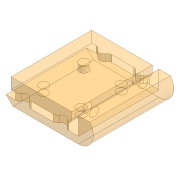
# Autodesk Inventor part: flange7-tip
Saved by Autodesk Inventor 2021 (Build 250183000, 183)
## iProperties
Created: 2022-10-18
Part Number: flange7-tip
Material: Rubber, Silicone
Document SubType Name: Modeling
Designer: alyn649
Density: 1.25 g/cm^3
Appearance: Clear - Yellow(1)
Author: alyn649
Autodesk Inventor part; units mm, degrees
ref_plane "YZ Plane" through (0, 0, 0) normal (1, 0, 0) x (0, 1, 0)
ref_plane "XZ Plane" through (0, 0, 0) normal (0, 1, 0) x (-1, 0, 0)
ref_plane "XY Plane" through (0, 0, 0) normal (0, 0, 1) x (1, 0, 0)
sketch "Sketch2" plane through (0, 0, 0) normal (0, 0, 1) x (1, 0, 0)
  line L0 (-8.072, 0) -> (8.072, 0)
  line L1 (8.072, -1.5) -> (-6.5187, -1.5)
  line L2 (-6.5187, -1.5) -> (-8.072, 0)
  line L3 (-8.8153, 7.7377) -> (-16.0231, 7.7377) construction
  line L4 (8.072, 0) -> (19.7494, 0) construction
  line L5 (8.072, 4) -> (8.072, 0)
  line L6 (8.072, 4) -> (12.608, 4) construction
  arc A0 (8.072, -1.5) -> (10.608, 4) centre (8.072, 1.8347) ccw
  line L7 (10.608, 4) -> (8.072, 4)
  point P0 (0, 0)
  point P1 (0, 0)
  dimension "d0" = 16.144
  dimension "d1" = 136
  dimension "d3" = 1.5
  dimension "d24" = 4
  dimension "d25" = 4.536
  dimension "d26" = 2
  constraints: 16 end point, 4 horizontal, 3 point on circle, 1 centre point, 1 coincident, 1 collinear, 1 midpoint, 1 parallel, 1 point on line, 1 tangent, 1 vertical, 1 vertical alignment
  measures "d0" distance of L0.start L0.end
  measures "d1" angle of L2 L3
  measures "d3" distance between parallel lines of L0 L1
  measures "d24" distance of L5.start L0.end
  measures "d25" distance of L5.start L6.end
  measures "d26" distance of L6.end A0.end
extrude "Extrusion1" add sketch "Sketch2" along normal mid plane 18
sketch "Sketch3" plane through (-8.072, 0, 9) normal (0, 1, 0) x (1, 0, 0)
  circle A0 centre (3.866, 13.5) radius 1
  line L0 (0, 18) -> (16.144, 18) construction
  circle A1 centre (3.866, 18) radius 1 construction
  arc A2 (3, 17.5) -> (2.1339, 18) centre (2.1339, 17) ccw
  arc A3 (3, 17.5) -> (4.732, 17.5) centre (3.866, 18) ccw
  arc A4 (5.5981, 18) -> (4.732, 17.5) centre (5.5981, 17) ccw
  line L1 (2.1339, 18) -> (8.6251, 18) construction
  line L2 (0, 18) -> (0, 0) projected
  line L3 (5.5981, 18) -> (2.1339, 18)
  circle A5 centre (12.279, 13.5) radius 1
  arc A6 (11.413, 17.5) -> (10.5469, 18) centre (10.5469, 17) ccw
  arc A7 (11.413, 17.5) -> (13.145, 17.5) centre (12.279, 18) ccw
  arc A8 (14.0111, 18) -> (13.145, 17.5) centre (14.0111, 17) ccw
  line L4 (14.0111, 18) -> (10.5469, 18)
  line L5 (10.5469, 18) -> (17.0381, 18) construction
  point P0 (8.072, 9)
  point P1 (5.5981, 18)
  point P2 (12.279, 18)
  dimension "d7" = 4.5
  dimension "d8" = 2
  dimension "d9" = 2
  dimension "d10" = 1
  dimension "d11" = 1
  dimension "d23" = 3.866
  dimension "d29" = 8.413
  constraints: 14 point on circle, 9 centre point, 8 end point, 8 tangent, 4 point on line, 1 collinear, 1 horizontal, 1 vertical alignment, 16 other
  measures "d7" vertical distance of A0.centre point (8.072, 9)
  measures "d8" diameter of A1
  measures "d9" diameter of A0
  measures "d10" radius of A2
  measures "d11" radius of A4
  measures "d23" distance from line of L2 A0.centre
  measures "d29" distance of A0.centre A5.centre
extrude "Extrusion2" add sketch "Sketch3" along normal blind 1.5
sketch "Sketch6" plane through (8.072, 4, -9) normal (-1, 0, 0) x (0, 0, 1)
  circle A0 centre (3.5, -1) radius 1
  line L0 (0, 0) -> (18, 0) projected
  line L1 (5.5, -2.5) -> (3.5, -2.5) projected
  point P0 (9, -4)
  point P1 (4.5, -2.5)
  dimension "d35" = 2
  dimension "d36" = 1
  constraints: 1 centre point, 1 midpoint, 1 tangent
  measures "d35" diameter of A0
  measures "d36" horizontal distance of point (4.5, -2.5) A0.centre
extrude "Extrusion5" add sketch "Sketch6" along normal blind 1.5
sketch "Sketch7" plane through (0, 0, -9) normal (0, 0, -1) x (-1, 0, 0)
  line L0 (-8.072, 4) -> (-10.608, 4) construction
  arc A0 (-10.608, 4) -> (-8.072, -1.5) centre (-8.072, 1.8347) ccw construction
  line L1 (-8.072, -1.5) -> (6.5187, -1.5) construction
  line L2 (6.5187, -1.5) -> (8.072, 0) construction
  line L3 (8.072, 0) -> (5.9381, 0) construction
  line L4 (5.9381, 0) -> (5.9381, 1.5) construction
  line L5 (2.4739, 1.5) -> (5.9381, 1.5) construction
  line L6 (2.4739, 0) -> (2.4739, 1.5) construction
  line L7 (2.4739, 0) -> (-2.4749, 0) construction
  line L8 (-2.4749, 0) -> (-2.4749, 1.5) construction
  line L9 (-5.9391, 1.5) -> (-2.4749, 1.5) construction
  line L10 (-5.9391, 0) -> (-5.9391, 1.5) construction
  line L11 (-5.9391, 0) -> (-8.072, 0) construction
  line L12 (-8.072, 0) -> (-8.072, 4) construction
  line L13 (-6.572, 2) -> (-6.572, 4) construction
  line L14 (-8.072, 4) -> (-8.072, 2) construction
  line L15 (-6.572, 4) -> (6.9381, 4)
  line L16 (6.9381, 4) -> (6.9381, 1.5)
  line L17 (6.9381, 1.5) -> (-6.572, 1.5)
  line L18 (-6.572, 1.5) -> (-6.572, 4)
  point P0 (0, 0)
  dimension "d39" = 1
  constraints: 8 end point, 2 parallel, 1 horizontal, 1 perpendicular, 1 point on line
  measures "d39" distance from line of L4.end L16
extrude "Extrusion6" add sketch "Sketch7" against normal blind 18
mirror "Mirror6" about plane through (0, 0, 0) normal (0, 0, 1) of "Extrusion5", "Extrusion2"
fillet "Fillet2" radius 1 1 edges at (6.572, 1.5, 0)
equation "\"d11\" = d10"
body "Solid1"
